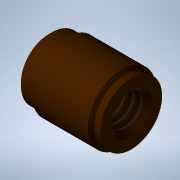
# Autodesk Inventor part: MBIS2-3-4
Saved by Autodesk Inventor 2021 (Build 250183000, 183)
## iProperties
Category: PARTsolutions
Company: MISUMI
Created: 2025-06-12
Part Number: MBIS2-3-4
Material: Generic
Catalog Web Link: www.cadenas.de
Description: MBIS-Brass Bit Insert Stand Type -Standard, One Sided-
Vendor: MISUMI
Document SubType Name: Modeling
Designer: psAdmin
Manufacturer: MISUMI
Mass: 0.0245587 g
Surface Area: 0.701657 cm^2
Volume: 0.0245587 cm^3
Density: 1 g/cm^3
Appearance: PSOLRGB-188-135-10
PSOL_IDENT_0: {$CADENAS_DATA/23d-libs/misumi/metric/28_keys_magnets/mbis.prj},157 {VTYP=3D},{NB=MBIS2-3-4},{LINA=M
PSOL_IDENT_1: BIS2-3-4},{NN=MBIS},{DATE=04.06.2021 05:54:11},{GEOMDATE=03.03.2020 00:37:47},{VERSION=},{LINEID=100
PSOL_IDENT_2: },{WBVAR=},{WBNUMERIC=}  {NB=MBIS2-3-4},{LINA=MBIS2-3-4},{KT=DUMMY},{PN=MBIS2-3-4},{TYPE=MBIS},{NO=2
PSOL_IDENT_3: -3-4},{M=2},{MP=M2x0.4},{D1=3.0},{D2=3.3},{L=4.0},{PITCH=0.40},{KNO=1.0},{D1L=0.30},{KL1=0.0},{KL2=3
PSOL_IDENT_4: .00},{KL3=0.0},{R=0.15}
NB: MBIS2-3-4
NN: MBIS
NT: Brass Bit Insert Stand Type -Standard, One Sided-
NBSYN: $PN.
LINA: MBIS2-3-4
CATALOG: Misumi
PN: MBIS2-3-4
TYPE: MBIS
NO: 2-3-4
M: 2
MP: M2x0.4
D1: 3
D2: 3.3
L: 4
SUPPLIER: MISUMI
ARTICLENO: MBIS2-3-4
BOMINFO: MBIS2-3-4
CREATOR: CADENAS GmbH
Title: MBIS2-3-4
Author: Cadenas PARTsolutions
Comments: Brass Bit Insert Stand Type -Standard, One Sided-
Autodesk Inventor part; units mm, degrees
ref_plane "YZ Plane" through (0, 0, 0) normal (1, 0, 0) x (0, 1, 0)
ref_plane "XZ Plane" through (0, 0, 0) normal (0, 1, 0) x (-1, 0, 0)
ref_plane "XY Plane" through (0, 0, 0) normal (0, 0, 1) x (1, 0, 0)
sketch "_____2" plane through (0, 0, 0) normal (0, 0, 1) x (1, 0, 0)
  line L0 (4, 0) -> (0, 0)
  line L1 (0, 0) -> (0, 1.35)
  line L2 (0, 1.35) -> (0.15, 1.5)
  line L3 (0.15, 1.5) -> (0.7, 1.5)
  line L4 (0.7, 1.5) -> (0.85, 1.65)
  line L5 (0.85, 1.65) -> (3.55, 1.65)
  line L6 (3.55, 1.65) -> (3.7, 1.5)
  line L7 (3.7, 1.5) -> (4, 1.5)
  line L8 (4, 1.5) -> (4, 0)
  line L9 (4, 0) -> (0, 0)
  constraints: 20 end point
revolve "Revolution1" add sketch "_____2" angle 360 about axis through (4, 0, 0) along (1, 0, 0)
sketch "Sketch2" plane through (4, 0, 0) normal (1, 0, 0) x (0, 0, -1)
  point P0 (0, 0)
hole "Hole1" at (4, 0, 0) direction (-1, 0, 0) diameter 1.567 depth 4 countersink diameter 2 countersink angle 90 thread size "M2x0.4" class "6H" standard "ISO Metric profile"
body "Solid1"
